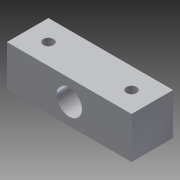
# Autodesk Inventor part: motormount
Saved by Autodesk Inventor 2013 (Build 170138000, 138)
## iProperties
Created: 2013-01-16
Part Number: motormount
Material: ABS Plastic
Document SubType Name: Modeling
Designer: geohot
Density: 1.06 g/cm^3
Mass: 5.66197 g
Surface Area: 26.9496 cm^2
Volume: 5.34148 cm^3
Author: geohot
Autodesk Inventor part; units mm, degrees
ref_plane "YZ Plane" through (0, 0, 0) normal (1, 0, 0) x (0, 1, 0)
ref_plane "XZ Plane" through (0, 0, 0) normal (0, 1, 0) x (-1, 0, 0)
ref_plane "XY Plane" through (0, 0, 0) normal (0, 0, 1) x (1, 0, 0)
sketch "Sketch1" plane through (0, 0, 0) normal (0, 0, 1) x (1, 0, 0)
  circle A0 centre (0, 0) radius 3.8862 projected
  line L0 (-19.05, 6.35) -> (19.05, 6.35)
  line L1 (19.05, 6.35) -> (19.05, -6.35)
  line L2 (19.05, -6.35) -> (-19.05, -6.35)
  line L3 (-19.05, -6.35) -> (-19.05, 6.35)
  point P0 (0, 0)
  dimension "d0" = 38.1
  dimension "d2" = 12.7
  dimension "d3" = 6.35
  dimension "d4" = 19.05
  constraints: 8 end point, 2 parallel, 1 horizontal, 1 perpendicular
  measures "d0" distance of L0.start L0.end
  measures "d2" distance of L0.end L1.end
  measures "d3" distance from line of L0 point (0, 0)
  measures "d4" distance from line of L3 point (0, 0)
extrude "Extrusion1" add sketch "Sketch1" against normal blind 12.7
sketch "Sketch2" plane through (-19.05, 6.35, 0) normal (0, 1, 0) x (1, 0, 0)
  line L0 (38.1, 0) -> (38.1, 12.7) projected
  line L1 (0, 0) -> (0, 12.7) projected
  circle A0 centre (6.35, 6.35) radius 1.5875
  circle A1 centre (31.75, 6.35) radius 1.5875
  point P0 (19.05, 0)
  dimension "d7" = 3.175
  dimension "d9" = 6.35
  dimension "d10" = 6.35
  constraints: 2 centre point, 1 equal radius
  measures "d7" diameter of A0
  measures "d9" distance from line of L1 A0.centre
  measures "d10" distance from line of L0 A1.centre
extrude "Extrusion2" cut sketch "Sketch2" against normal up to next
body "Solid1"
